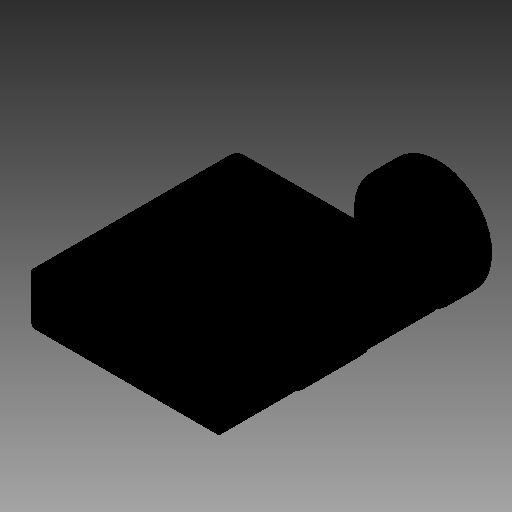
# Autodesk Inventor part: 4489_a
Saved by Autodesk Inventor 2019 (Build 230136000, 136)
## iProperties
Category: PARTsolutions
Company: 8020
Created: 2019-03-04
Part Number: 4489_a
Material: Generic
Catalog Web Link: www.cadenas.de
Description: 4488, 4489_a-Combination Hinges
Vendor: 8020
Document SubType Name: Modeling
Designer: psadmin
Manufacturer: 8020
Mass: 14.2057 g
Surface Area: 62.5163 cm^2
Volume: 14.2057 cm^3
Density: 1 g/cm^3
Appearance: PSOLRGB-0-0-0
PSOL_IDENT_0: {$CADENAS_DATA\23d-libs\8020\inch\panels_and_doors\4488_a.prj},160 {VTYP=3D},{NB=4489_a},{LINA=4489_
PSOL_IDENT_1: a},{NN=4488, 4489_a},{DATE=04.12.2018 10:30:19},{GEOMDATE=03.01.2012 08:02:00},{VERSION=},{LINEID=10
PSOL_IDENT_2: },{WBVAR=TS},{WBNUMERIC=}  {NB=4489_a},{LINA=4489_a},{KT=DUMMY},{PN=4489},{TS=Without Handle},{A=2.9
PSOL_IDENT_3: 1338583},{B=1.57480315},{C=0.82677165},{D=1.77165354},{E=0.88582677},{F=N/A},{F1=0.00000000},{G=0.95
PSOL_IDENT_4: 400000},{H=0.56200000},{J=N/A},{J1=0.00000000},{K=0.31199999},{L=0.27200000},{M=0.32283465},{W=.42}
NN: 4488, 4489_a
NT: Combination Hinges
NB: 4489_a
NBSYN: $PN._a
LINA: 4489_a
PN: 4489
TS: Without Handle
A: 2.91338583
B: 1.57480315
C: 0.82677165
D: 1.77165354
E: 0.88582677
F: N/A
G: 0.954
H: 0.562
J: N/A
K: 0.31199999
L: 0.272
M: 0.32283465
W: .42
SUPPLIER: 8020
ARTICLENO: 4489_a
BOMINFO: 4489_a
CREATOR: CADENAS GmbH
Title: 4489_a
Author: Cadenas PARTsolutions
Comments: Combination Hinges
Autodesk Inventor part; units mm, degrees
sketch "Sketch_1" plane through (0, 0, 0) normal (0, 1, 0) x (-1, 0, 0)
  arc A0 (37, 16) -> (33, 20) centre (33, 16) ccw
  line L0 (33, 20) -> (0.6018, 20)
  line L1 (0.6018, 20) -> (0.6018, -20)
  line L2 (0.6018, -20) -> (33, -20)
  arc A1 (33, -20) -> (37, -16) centre (33, -16) ccw
  line L3 (37, -16) -> (37, 16)
  circle A2 centre (22.5, 10.5) radius 4.1
  circle A3 centre (22.5, -10.5) radius 4.1
  constraints: 8 end point, 4 centre point, 4 point on circle
extrude "Extrusion1" add sketch "Sketch_1" along normal blind 7.9248
sketch "Sketch_2" plane through (0, 0, 0) normal (0, 0, 1) x (1, 0, 0)
  line L0 (-74, 15.8496) -> (-74, -7.9248)
  line L1 (-74, -7.9248) -> (37, -7.9248)
  line L2 (37, -7.9248) -> (37, 15.8496)
  line L3 (37, 15.8496) -> (-74, 15.8496)
  arc A0 (-37, 0.5) -> (-36.5, 0) centre (-36.5, 0.5) ccw
  line L4 (-36.5, 0) -> (-0.6, 0)
  line L5 (-0.6, 0) -> (-0.6, 7.9248)
  line L6 (-0.6, 7.9248) -> (-35.5, 7.9248)
  arc A1 (-35.5, 7.9248) -> (-37, 6.4248) centre (-35.5, 6.4248) ccw
  line L7 (-37, 6.4248) -> (-37, 0.5)
  constraints: 16 end point, 4 point on circle, 2 centre point
extrude "Extrusion2" cut sketch "Sketch_2" along normal mid plane 40
sketch "Sketch_3" plane through (0, 0, 0) normal (1, 0, 0) x (0, 1, 0)
  line L0 (15.8496, 40) -> (-7.9248, 40)
  line L1 (-7.9248, 40) -> (-7.9248, -40)
  line L2 (-7.9248, -40) -> (15.8496, -40)
  line L3 (15.8496, -40) -> (15.8496, 40)
  arc A0 (0.5, 20) -> (0, 19.5) centre (0.5, 19.5) ccw
  line L4 (0, 19.5) -> (0, -19.5)
  arc A1 (0, -19.5) -> (0.5, -20) centre (0.5, -19.5) ccw
  line L5 (0.5, -20) -> (6.4248, -20)
  arc A2 (6.4248, -20) -> (7.9248, -18.5) centre (6.4248, -18.5) ccw
  line L6 (7.9248, -18.5) -> (7.9248, 18.5)
  arc A3 (7.9248, 18.5) -> (6.4248, 20) centre (6.4248, 18.5) ccw
  line L7 (6.4248, 20) -> (0.5, 20)
  constraints: 16 end point, 8 point on circle, 4 centre point
extrude "Extrusion3" cut sketch "Sketch_3" against normal blind 74
sketch "Sketch_4" plane through (0, 0, 0) normal (0, 0, 1) x (1, 0, 0)
  circle A0 centre (0, 14.2748) radius 10.5
  constraints: 1 centre point
extrude "Extrusion4" cut sketch "Sketch_4" along normal mid plane 40
sketch "Sketch_5" plane through (0, 14.2748, 0) normal (0, 1, 0) x (1, 0, 0)
  arc A0 (-9.9568, -11.5) -> (-9.4568, -12) centre (-9.4568, -11.5) ccw
  line L0 (-9.4568, -12) -> (-0.6018, -12)
  line L1 (-0.6018, -12) -> (-0.6018, -1)
  line L2 (-0.6018, -1) -> (-9.4568, -1)
  arc A1 (-9.4568, -1) -> (-9.9568, -1.5) centre (-9.4568, -1.5) ccw
  line L3 (-9.9568, -1.5) -> (-9.9568, -11.5)
  constraints: 8 end point, 4 point on circle, 2 centre point
extrude "Extrusion5" add sketch "Sketch_5" against normal blind 11.7348
sketch "Sketch_6" plane through (0, 14.2748, 0) normal (0, 1, 0) x (1, 0, 0)
  line L0 (0, -1) -> (0, -12)
  line L1 (0, -12) -> (-9.4568, -12)
  arc A0 (-9.9568, -11.5) -> (-9.4568, -12) centre (-9.4568, -11.5) ccw
  line L2 (-9.9568, -11.5) -> (-9.9568, -1.5)
  arc A1 (-9.4568, -1) -> (-9.9568, -1.5) centre (-9.4568, -1.5) ccw
  line L3 (-9.4568, -1) -> (0, -1)
  line L4 (0, -1) -> (0, -12)
  constraints: 10 end point, 4 point on circle, 2 centre point
revolve "Revolution1" add sketch "Sketch_6" angle 360 about axis through (0, 14.2748, 1) along (0, 0, -1)
sketch "Sketch_7" plane through (0, 14.2748, 0) normal (0, 1, 0) x (1, 0, 0)
  arc A0 (-9.9568, 14.5) -> (-9.4568, 14) centre (-9.4568, 14.5) ccw
  line L0 (-9.4568, 14) -> (-0.6018, 14)
  line L1 (-0.6018, 14) -> (-0.6018, 20)
  line L2 (-0.6018, 20) -> (-9.4568, 20)
  arc A1 (-9.4568, 20) -> (-9.9568, 19.5) centre (-9.4568, 19.5) ccw
  line L3 (-9.9568, 19.5) -> (-9.9568, 14.5)
  constraints: 8 end point, 4 point on circle, 2 centre point
extrude "Extrusion6" add sketch "Sketch_7" against normal blind 11.7348
sketch "Sketch_8" plane through (0, 14.2748, 0) normal (0, 1, 0) x (1, 0, 0)
  line L0 (0, 20) -> (0, 14)
  line L1 (0, 14) -> (-9.4568, 14)
  arc A0 (-9.9568, 14.5) -> (-9.4568, 14) centre (-9.4568, 14.5) ccw
  line L2 (-9.9568, 14.5) -> (-9.9568, 19.5)
  arc A1 (-9.4568, 20) -> (-9.9568, 19.5) centre (-9.4568, 19.5) ccw
  line L3 (-9.4568, 20) -> (0, 20)
  line L4 (0, 20) -> (0, 14)
  constraints: 10 end point, 4 point on circle, 2 centre point
revolve "Revolution2" add sketch "Sketch_8" angle 360 about axis through (0, 14.2748, -20) along (0, 0, -1)
sketch "Sketch_9" plane through (0, 0, 0) normal (0, 0, 1) x (1, 0, 0)
  circle A0 centre (0, 14.2748) radius 4.25
  constraints: 1 centre point
extrude "Extrusion7" cut sketch "Sketch_9" along normal mid plane 40
ref_plane "to_b_XY" through (0, 14.2748, 0) normal (0, 0, -1) x (1, 0, 0)
ref_plane "to_b_YZ" through (0, 14.2748, 0) normal (1, 0, 0) x (0, -1, 0)
ref_plane "to_b_ZX" through (0, 14.2748, 0) normal (0, -1, 0) x (0, 0, -1)
ref_plane "to_pin_XY" through (0, 14.2748, 0) normal (0, 0, 1) x (1, 0, 0)
ref_plane "to_pin_YZ" through (0, 14.2748, 0) normal (1, 0, 0) x (0, 1, 0)
ref_plane "to_pin_ZX" through (0, 14.2748, 0) normal (0, 1, 0) x (0, 0, 1)
ref_plane "to_washer1_XY" through (0, 14.2748, 12.1745) normal (0, 0, -1) x (1, 0, 0)
ref_plane "to_washer1_YZ" through (0, 14.2748, 12.1745) normal (1, 0, 0) x (0, -1, 0)
ref_plane "to_washer1_ZX" through (0, 14.2748, 12.1745) normal (0, -1, 0) x (0, 0, -1)
ref_plane "to_washer2_XY" through (0, 14.2748, 0.8255) normal (0, 0, 1) x (1, 0, 0)
ref_plane "to_washer2_YZ" through (0, 14.2748, 0.8255) normal (1, 0, 0) x (0, 1, 0)
ref_plane "to_washer2_ZX" through (0, 14.2748, 0.8255) normal (0, 1, 0) x (0, 0, 1)
ref_plane "to_washer3_XY" through (0, 14.2748, -13.8255) normal (0, 0, -1) x (1, 0, 0)
ref_plane "to_washer3_YZ" through (0, 14.2748, -13.8255) normal (1, 0, 0) x (0, -1, 0)
ref_plane "to_washer3_ZX" through (0, 14.2748, -13.8255) normal (0, -1, 0) x (0, 0, -1)
body "Solid1"
